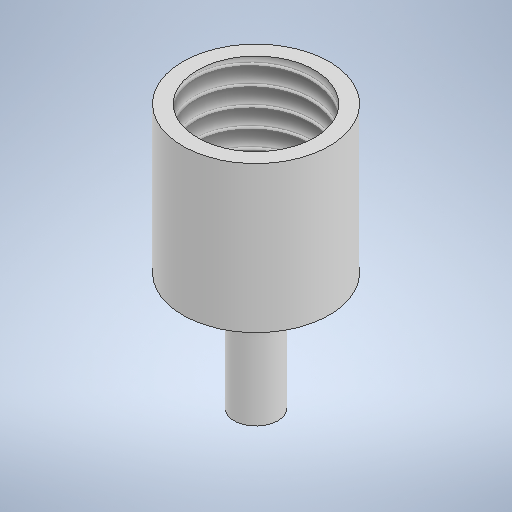
# Autodesk Inventor part: Part9
Saved by Autodesk Inventor 2025 (Build 290162000, 162)
## iProperties
Created: 2026-06-20
Part Number: Part9
Material: Generic
Document SubType Name: Modeling
Designer: saket
Density: 1 g/cm^3
Appearance: Default
Author: saket
Autodesk Inventor part; units mm, degrees
ref_plane "YZ Plane" through (0, 0, 0) normal (1, 0, 0) x (0, 1, 0)
ref_plane "XZ Plane" through (0, 0, 0) normal (0, 1, 0) x (-1, 0, 0)
ref_plane "XY Plane" through (0, 0, 0) normal (0, 0, 1) x (1, 0, 0)
sketch "Sketch1" plane through (0, 0, 0) normal (0, 1, 0) x (-1, 0, 0)
  circle A0 centre (0, 0) radius 4
  circle A1 centre (0, 0) radius 5
  circle A2 centre (0, 0) radius 1
  circle A3 centre (0, 0) radius 1.5
  dimension "d0" = 8
  dimension "d1" = 10
  dimension "d2" = 2
  dimension "d3" = 3
  constraints: 4 centre point, 4 coincident
  measures "d0" diameter of A0
  measures "d1" diameter of A1
  measures "d2" diameter of A2
  measures "d3" diameter of A3
extrude "Extrusion1" add sketch "Sketch1" along normal blind 10 contours A1
extrude "Extrusion2" add sketch "Sketch1" along normal blind 4 contours A0 | A3
extrude "Extrusion3" add sketch "Sketch1" against normal blind 8 contours A3
thread "Thread1" size "M8x1.25" class "6H" standard "ANSI Metric M Profile" length 10
body "Solid1"
